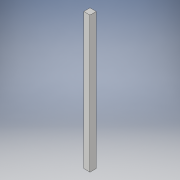
# Autodesk Inventor part: HeaderPin
Saved by Autodesk Inventor 2019 (Build 230136000, 136)
## iProperties
Created: 2019-07-16
Part Number: HeaderPin
Material: Generic
Document SubType Name: Modeling
Designer: james
Density: 1 g/cm^3
Appearance: Default
Author: james
Autodesk Inventor part; units mm, degrees
ref_plane "YZ Plane" through (0, 0, 0) normal (1, 0, 0) x (0, 1, 0)
ref_plane "XZ Plane" through (0, 0, 0) normal (0, 1, 0) x (-1, 0, 0)
ref_plane "XY Plane" through (0, 0, 0) normal (0, 0, 1) x (1, 0, 0)
sketch "Sketch1" plane through (0, 0, 0) normal (1, 0, 0) x (0, 1, 0)
  line L0 (5.6299, 7.769) -> (-7.9101, 7.769)
  line L1 (-7.9101, 7.769) -> (-7.9101, 7.149)
  line L2 (-7.9101, 7.149) -> (5.6299, 7.149)
  line L3 (5.6299, 7.149) -> (5.6299, 7.769)
  point P0 (0, 0)
  dimension "d0" = 13.54
  dimension "d1" = 0.62
  constraints: 8 end point, 2 parallel, 1 horizontal, 1 perpendicular
  measures "d0" distance of L0.start L0.end
  measures "d1" distance of L0.end L1.end
extrude "Extrusion1" add sketch "Sketch1" along normal blind 0.62
body "Solid1"
